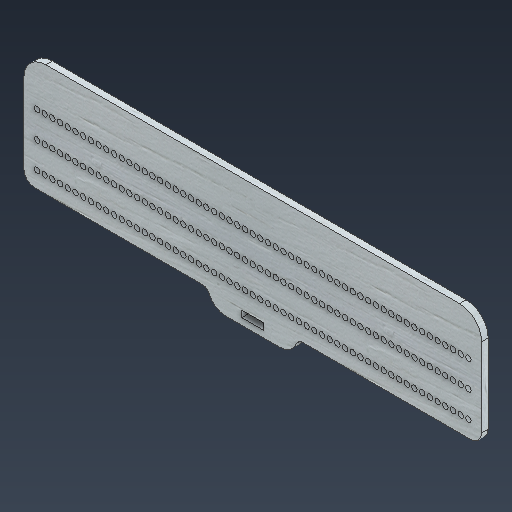
# Autodesk Inventor part: side_frame_test
Saved by Autodesk Inventor 2025.3 (Build 293356030, 356C)
## iProperties
Created: 2025-09-04
Part Number: side_frame_test
Material: 木材 (楓木)
Document SubType Name: Modeling
Designer: 陳泓任
Density: 0.67 g/cm^3
Appearance: 木材 - 白色刷漆
Author: 陳泓任
Autodesk Inventor part; units mm, degrees
ref_plane "YZ Plane" through (0, 0, 0) normal (1, 0, 0) x (0, 1, 0)
ref_plane "XZ Plane" through (0, 0, 0) normal (0, 1, 0) x (-1, 0, 0)
ref_plane "XY Plane" through (0, 0, 0) normal (0, 0, 1) x (1, 0, 0)
sketch "草圖1" plane through (0, 0, 0) normal (0, 0, 1) x (1, 0, 0)
  arc A0 (99, -19.3985) -> (104, -14.3985) centre (99, -14.3985) ccw
  arc A1 (-104, -14.3985) -> (-99, -19.3985) centre (-99, -14.3985) ccw
  circle A2 centre (0, 12) radius 1.25
  circle A3 centre (0, -12) radius 1.25
  line L0 (-99, -19.3985) -> (-22.615, -19.3985)
  arc A4 (22.615, -19.3985) -> (19.8099, -21.3349) centre (22.615, -22.3985) ccw
  line L1 (-5, -23.4985) -> (-5, -20.4985)
  line L2 (-5, -20.4985) -> (5, -20.4985)
  line L3 (5, -20.4985) -> (5, -23.4985)
  line L4 (5, -23.4985) -> (-5, -23.4985)
  arc A5 (-19.8099, -21.3349) -> (-22.615, -19.3985) centre (-22.615, -22.3985) ccw
  line L5 (-12.3296, -26.4985) -> (12.3296, -26.4985)
  line L6 (22.615, -19.3985) -> (99, -19.3985)
  line L7 (0, -30.8826) -> (0, 56.0191) construction
  line L8 (-104.9871, 0) -> (119.3176, 0) construction
  line L9 (0, 12) -> (0, -12)
  circle A6 centre (3.5, 12) radius 1.25
  circle A7 centre (3.5, -12) radius 1.25
  circle A8 centre (-3.5, 12) radius 1.25
  circle A9 centre (-3.5, -12) radius 1.25
  circle A10 centre (7, 12) radius 1.25
  circle A11 centre (7, -12) radius 1.25
  circle A12 centre (-7, 12) radius 1.25
  circle A13 centre (-7, -12) radius 1.25
  circle A14 centre (10.5, 12) radius 1.25
  circle A15 centre (10.5, -12) radius 1.25
  circle A16 centre (-10.5, 12) radius 1.25
  circle A17 centre (-10.5, -12) radius 1.25
  circle A18 centre (14, 12) radius 1.25
  circle A19 centre (14, -12) radius 1.25
  circle A20 centre (-14, 12) radius 1.25
  circle A21 centre (-14, -12) radius 1.25
  circle A22 centre (17.5, 12) radius 1.25
  circle A23 centre (17.5, -12) radius 1.25
  circle A24 centre (-17.5, 12) radius 1.25
  circle A25 centre (-17.5, -12) radius 1.25
  circle A26 centre (21, 12) radius 1.25
  circle A27 centre (21, -12) radius 1.25
  circle A28 centre (-21, 12) radius 1.25
  circle A29 centre (-21, -12) radius 1.25
  circle A30 centre (24.5, 12) radius 1.25
  circle A31 centre (24.5, -12) radius 1.25
  circle A32 centre (-24.5, 12) radius 1.25
  circle A33 centre (-24.5, -12) radius 1.25
  circle A34 centre (28, 12) radius 1.25
  circle A35 centre (28, -12) radius 1.25
  circle A36 centre (-28, 12) radius 1.25
  circle A37 centre (-28, -12) radius 1.25
  circle A38 centre (31.5, 12) radius 1.25
  circle A39 centre (31.5, -12) radius 1.25
  circle A40 centre (-31.5, 12) radius 1.25
  circle A41 centre (-31.5, -12) radius 1.25
  circle A42 centre (35, 12) radius 1.25
  circle A43 centre (35, -12) radius 1.25
  circle A44 centre (-35, 12) radius 1.25
  circle A45 centre (-35, -12) radius 1.25
  circle A46 centre (38.5, 12) radius 1.25
  circle A47 centre (38.5, -12) radius 1.25
  circle A48 centre (-38.5, 12) radius 1.25
  circle A49 centre (-38.5, -12) radius 1.25
  circle A50 centre (42, 12) radius 1.25
  circle A51 centre (42, -12) radius 1.25
  circle A52 centre (-42, 12) radius 1.25
  circle A53 centre (-42, -12) radius 1.25
  circle A54 centre (45.5, 12) radius 1.25
  circle A55 centre (45.5, -12) radius 1.25
  circle A56 centre (-45.5, 12) radius 1.25
  circle A57 centre (-45.5, -12) radius 1.25
  circle A58 centre (49, 12) radius 1.25
  circle A59 centre (49, -12) radius 1.25
  circle A60 centre (-49, 12) radius 1.25
  circle A61 centre (-49, -12) radius 1.25
  circle A62 centre (52.5, 12) radius 1.25
  circle A63 centre (52.5, -12) radius 1.25
  circle A64 centre (-52.5, 12) radius 1.25
  circle A65 centre (-52.5, -12) radius 1.25
  circle A66 centre (56, 12) radius 1.25
  circle A67 centre (56, -12) radius 1.25
  circle A68 centre (-56, 12) radius 1.25
  circle A69 centre (-56, -12) radius 1.25
  circle A70 centre (59.5, 12) radius 1.25
  circle A71 centre (59.5, -12) radius 1.25
  circle A72 centre (-59.5, 12) radius 1.25
  circle A73 centre (-59.5, -12) radius 1.25
  circle A74 centre (63, 12) radius 1.25
  circle A75 centre (63, -12) radius 1.25
  circle A76 centre (-63, 12) radius 1.25
  circle A77 centre (-63, -12) radius 1.25
  circle A78 centre (66.5, 12) radius 1.25
  circle A79 centre (66.5, -12) radius 1.25
  circle A80 centre (-66.5, 12) radius 1.25
  circle A81 centre (-66.5, -12) radius 1.25
  circle A82 centre (70, 12) radius 1.25
  circle A83 centre (70, -12) radius 1.25
  circle A84 centre (-70, 12) radius 1.25
  circle A85 centre (-70, -12) radius 1.25
  circle A86 centre (73.5, 12) radius 1.25
  circle A87 centre (73.5, -12) radius 1.25
  circle A88 centre (-73.5, 12) radius 1.25
  circle A89 centre (-73.5, -12) radius 1.25
  circle A90 centre (77, 12) radius 1.25
  circle A91 centre (77, -12) radius 1.25
  circle A92 centre (-77, 12) radius 1.25
  circle A93 centre (-77, -12) radius 1.25
  circle A94 centre (80.5, 12) radius 1.25
  circle A95 centre (80.5, -12) radius 1.25
  circle A96 centre (-80.5, 12) radius 1.25
  circle A97 centre (-80.5, -12) radius 1.25
  circle A98 centre (84, 12) radius 1.25
  circle A99 centre (84, -12) radius 1.25
  circle A100 centre (-84, 12) radius 1.25
  circle A101 centre (-84, -12) radius 1.25
  circle A102 centre (87.5, 12) radius 1.25
  circle A103 centre (87.5, -12) radius 1.25
  circle A104 centre (-87.5, 12) radius 1.25
  circle A105 centre (-87.5, -12) radius 1.25
  circle A106 centre (91, 12) radius 1.25
  circle A107 centre (91, -12) radius 1.25
  circle A108 centre (-91, 12) radius 1.25
  circle A109 centre (-91, -12) radius 1.25
  circle A110 centre (94.5, 12) radius 1.25
  circle A111 centre (94.5, -12) radius 1.25
  circle A112 centre (-94.5, 12) radius 1.25
  circle A113 centre (-94.5, -12) radius 1.25
  circle A114 centre (98, 12) radius 1.25
  circle A115 centre (98, -12) radius 1.25
  circle A116 centre (-98, 12) radius 1.25
  circle A117 centre (-98, -12) radius 1.25
  line L10 (-94, 31.5) -> (94, 31.5)
  line L11 (-104, -14.3985) -> (-104, 21.5)
  line L12 (104, 21.5) -> (104, -14.3985)
  arc A118 (-94, 31.5) -> (-104, 21.5) centre (-94, 21.5) ccw
  arc A119 (104, 21.5) -> (94, 31.5) centre (94, 21.5) ccw
  circle A120 centre (0, 0) radius 1.25
  circle A121 centre (7, 0) radius 1.25
  circle A122 centre (10.5, 0) radius 1.25
  circle A123 centre (14, 0) radius 1.25
  circle A124 centre (-3.5, 0) radius 1.25
  circle A125 centre (3.5, 0) radius 1.25
  circle A126 centre (-21, 0) radius 1.25
  circle A127 centre (-17.5, 0) radius 1.25
  circle A128 centre (-14, 0) radius 1.25
  circle A129 centre (-7, 0) radius 1.25
  circle A130 centre (17.5, 0) radius 1.25
  circle A131 centre (21, 0) radius 1.25
  circle A132 centre (24.5, 0) radius 1.25
  circle A133 centre (28, 0) radius 1.25
  circle A134 centre (31.5, 0) radius 1.25
  circle A135 centre (38.5, 0) radius 1.25
  circle A136 centre (42, 0) radius 1.25
  circle A137 centre (45.5, 0) radius 1.25
  circle A138 centre (35, 0) radius 1.25
  circle A139 centre (49, 0) radius 1.25
  circle A140 centre (52.5, 0) radius 1.25
  circle A141 centre (56, 0) radius 1.25
  circle A142 centre (59.5, 0) radius 1.25
  circle A143 centre (63, 0) radius 1.25
  circle A144 centre (66.5, 0) radius 1.25
  circle A145 centre (70, 0) radius 1.25
  circle A146 centre (77, 0) radius 1.25
  circle A147 centre (80.5, 0) radius 1.25
  circle A148 centre (84, 0) radius 1.25
  circle A149 centre (87.5, 0) radius 1.25
  circle A150 centre (91, 0) radius 1.25
  circle A151 centre (94.5, 0) radius 1.25
  circle A152 centre (98, 0) radius 1.25
  circle A153 centre (73.5, 0) radius 1.25
  circle A154 centre (-10.5, 0) radius 1.25
  circle A155 centre (-28, 0) radius 1.25
  circle A156 centre (-31.5, 0) radius 1.25
  circle A157 centre (-24.5, 0) radius 1.25
  circle A158 centre (-35, 0) radius 1.25
  circle A159 centre (-38.5, 0) radius 1.25
  circle A160 centre (-42, 0) radius 1.25
  circle A161 centre (-45.5, 0) radius 1.25
  circle A162 centre (-49, 0) radius 1.25
  circle A163 centre (-52.5, 0) radius 1.25
  circle A164 centre (-59.5, 0) radius 1.25
  circle A165 centre (-63, 0) radius 1.25
  circle A166 centre (-56, 0) radius 1.25
  circle A167 centre (-70, 0) radius 1.25
  circle A168 centre (-73.5, 0) radius 1.25
  circle A169 centre (-77, 0) radius 1.25
  circle A170 centre (-80.5, 0) radius 1.25
  circle A171 centre (-84, 0) radius 1.25
  circle A172 centre (-87.5, 0) radius 1.25
  circle A173 centre (-91, 0) radius 1.25
  circle A174 centre (-66.5, 0) radius 1.25
  circle A175 centre (-94.5, 0) radius 1.25
  circle A176 centre (-98, 0) radius 1.25
  arc A177 (-19.8099, -21.3349) -> (-12.3296, -26.4985) centre (-12.3296, -18.4985) ccw
  arc A178 (12.3296, -26.4985) -> (19.8099, -21.3349) centre (12.3296, -18.4985) ccw
  line L13 (-10.7829, -20.4005) -> (9.25, -20.4005) construction
  point P0 (0, 0)
  point P1 (0, -20.4985)
  dimension "d0" = 10
  dimension "d1" = 3
  dimension "d2" = 3
  dimension "d4" = 2.5
  dimension "d12" = 3
  dimension "d29" = 45.23
  dimension "d92" = 3.5
  dimension "d97" = 7.3985
  dimension "d98" = 5
  dimension "d100" = 208
  dimension "d101" = 19.5
  dimension "d102" = 10
  dimension "d131" = 12
  dimension "d137" = 12
  dimension "d138" = 8
  dimension "d139" = 7.1
  constraints: 179 centre point, 28 end point, 16 point on circle, 14 tangent, 7 horizontal, 4 equal radius, 4 vertical, 3 perpendicular, 3 point on line, 2 collinear, 1 midpoint, 341 other
  measures "d0" distance of L3.end L1.start
  measures "d1" distance of L1.start L1.end
  measures "d2" distance between parallel lines of L5 L4
  measures "d4" diameter of A2
  measures "d12" radius of A5
  measures "d29" distance of A4.centre A5.centre
  measures "d92" distance of L9.start A6.centre
  measures "d97" distance from line of L6 A107.centre
  measures "d98" radius of A1
  measures "d100" diameter of L11 L7
  measures "d101" distance from line of L10 A102.centre
  measures "d102" radius of A118
  measures "d131" distance of L9.start A120.centre
  measures "d137" distance of L9.end A120.centre
  measures "d138" radius of A177
  measures "d139" distance between parallel lines of L0 L5
extrude "擠出1" add sketch "草圖1" along normal mid plane 3
sketch "草圖3" plane through (0, 0, 1.5) normal (0, 0, 1) x (1, 0, 0)
  line L0 (0, 52.3829) -> (0, -39.0235)
  line L1 (-112.5881, 0) -> (123.4866, 0)
  point P0 (0, 0)
  constraints: 4 end point, 2 point on line, 1 horizontal, 1 vertical
